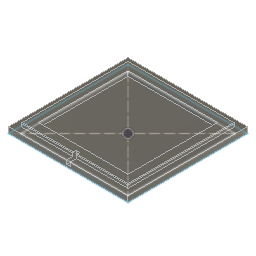
Cover Silicone Container (Autodesk Fusion 360 design; units mm, degrees)
Autodesk Fusion 360 part; units mm, degrees
sketch "Sketch1" plane through (0, 0, 0) normal (0, 0, 1) x (1, 0, 0)
  line L0 (50, 50) -> (-50, 50)
  line L1 (-50, 50) -> (-50, -50)
  line L2 (-50, -50) -> (50, -50)
  line L3 (50, -50) -> (50, 50)
  line L4 (50, 50) -> (-50, -50) construction
  line L5 (-50, 50) -> (50, -50) construction
  line L6 (44.75, 44.75) -> (-44.75, 44.75)
  line L7 (-44.75, 44.75) -> (-44.75, -44.75)
  line L8 (-44.75, -44.75) -> (44.75, -44.75)
  line L9 (44.75, -44.75) -> (44.75, 44.75)
  line L10 (44.75, 44.75) -> (-44.75, -44.75) construction
  line L11 (-44.75, 44.75) -> (44.75, -44.75) construction
  dimension "d1" = 89.5
  dimension "d12" = 89.5
  constraint horizontal L0
  constraint perpendicular L0 L1
  constraint parallel L0 L2
  constraint parallel L1 L3
  constraint coincident L4 origin
  constraint coincident L5 origin
  constraint horizontal L6
  constraint perpendicular L6 L7
  constraint parallel L6 L8
  constraint parallel L7 L9
  constraint coincident L10 origin
  constraint coincident L11 origin
  measures "d1" distance of L6.end L7.end
  measures "d12" distance of L6.start L6.end
extrude "Extrude1" add sketch "Sketch1" along normal blind 5
extrude "Extrude2" add sketch "Sketch1" along normal blind 8 contours L6 L7 L8 L9
sketch "Sketch2" plane through (0, -50, 0) normal (0, -1, 0) x (1, 0, 0)
  line L0 (-50, 0) -> (50, 0)
  line L1 (50, 0) -> (50, 5)
  line L2 (50, 5) -> (-50, 5)
  line L3 (-50, 5) -> (-50, 0)
  line L4 (1.5, 8) -> (-1.5, 8)
  line L5 (-1.5, 8) -> (-1.5, 2)
  line L6 (-1.5, 2) -> (1.5, 2)
  line L7 (1.5, 2) -> (1.5, 8)
  line L8 (1.5, 8) -> (-1.5, 2) construction
  line L9 (-1.5, 8) -> (1.5, 2) construction
  point P0 (0, 5)
  dimension "d6" = 6
  dimension "d7" = 3
  constraint horizontal L4
  constraint perpendicular L4 L5
  constraint parallel L4 L6
  constraint parallel L5 L7
  constraint coincident L8 P0
  constraint coincident L9 P0
  constraint midpoint L2 P0
  measures "d6" distance of L4.end L5.end
  measures "d7" distance of L5.end L6.end
extrude "Extrude3" cut sketch "Sketch2" against normal blind 8 contours L2 L4 L5 L7 | L2 L5 L6 L7
chamfer "Chamfer1" distance 0.5 angle 45 4 edges at (-23.125, -44.75, 8) (-44.75, 0, 8) (23.125, -44.75, 8) (44.75, 0, 8)
chamfer "Chamfer1" distance 0.5 angle 45 1 edges at (0, 44.75, 8)
sketch "Sketch3" plane through (0, 0, 8) normal (0, 0, 1) x (-1, 0, 0)
  line L0 (44.25, 44.25) -> (1.5, 44.25)
  line L1 (1.5, 44.25) -> (1.5, 42)
  line L2 (1.5, 42) -> (-1.5, 42)
  line L3 (-1.5, 42) -> (-1.5, 44.25)
  line L4 (-1.5, 44.25) -> (-44.25, 44.25)
  line L5 (-44.25, 44.25) -> (-44.25, -44.25)
  line L6 (-44.25, -44.25) -> (44.25, -44.25)
  line L7 (44.25, -44.25) -> (44.25, 44.25)
  line L8 (-37.5, -37.5) -> (37.5, -37.5)
  line L9 (37.5, -37.5) -> (37.5, 37.5)
  line L10 (37.5, 37.5) -> (-37.5, 37.5)
  line L11 (-37.5, 37.5) -> (-37.5, -37.5)
  line L12 (-37.5, -37.5) -> (37.5, 37.5) construction
  line L13 (37.5, -37.5) -> (-37.5, 37.5) construction
  dimension "d13" = 75
  dimension "d14" = 75
  constraint horizontal L8
  constraint perpendicular L8 L9
  constraint parallel L8 L10
  constraint parallel L9 L11
  constraint coincident L12 origin
  constraint coincident L13 origin
  measures "d13" distance of L8.start L10.end
  measures "d14" distance of L8.start L8.end
extrude "Extrude4" cut sketch "Sketch3" against normal blind 4 contours L8 L9 L10 L11
